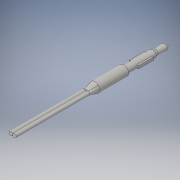
# Autodesk Inventor part: Snap-Twist Idea M
Saved by Autodesk Inventor 2016 (Build 200138000, 138)
## iProperties
Created: 2015-07-29
Part Number: Snap-Twist Idea M
Material: Generic
Document SubType Name: Modeling
Designer: Nancy
Density: 1 g/cm^3
Appearance: Default
Mass: 0.234963 g
Surface Area: 4.60785 cm^2
Volume: 0.234963 cm^3
Author: Nancy
Autodesk Inventor part; units mm, degrees
sketch "Sketch1" plane through (0, 0, 0) normal (0, 0, 1) x (1, 0, 0)
  circle A0 centre (0, 0) radius 0.3405
  dimension "d0" = 0.681
  constraints: 1 centre point, 1 coincident
  measures "d0" diameter of A0
ref_plane "Work Plane1" through (0, 0, 1) normal (0, 0, 1) x (1, 0, 0)
sketch "Sketch2" plane through (0, 0, 1) normal (0, 0, 1) x (1, 0, 0)
  circle A0 centre (0, 0) radius 1.0215
  dimension "d2" = 2.043
  constraints: 1 centre point, 1 coincident
  measures "d2" diameter of A0
ref_plane "Work Plane2" through (0, 0, 4) normal (0, 0, 1) x (1, 0, 0)
sketch "Sketch3" plane through (0, 0, 4) normal (0, 0, 1) x (1, 0, 0)
  circle A0 centre (0, 0) radius 0.8476
  dimension "d4" = 1.6951
  constraints: 1 centre point, 1 coincident
  measures "d4" diameter of A0
ref_plane "Work Plane3" through (0, 0, 5) normal (0, 0, 1) x (1, 0, 0)
sketch "Sketch4" plane through (0, 0, 5) normal (0, 0, 1) x (1, 0, 0)
  circle A0 centre (0, 0) radius 1.1935
  dimension "d6" = 2.387
  constraints: 1 centre point, 1 coincident
  measures "d6" diameter of A0
loft "Loft1" add profiles "Sketch4", "Sketch3"
loft "Loft2" add profiles "Sketch2" section 1 edges at (-0.8476, 0, 4)
loft "Loft3" add profiles "Sketch1" section 2 edges at (-1.0215, 0, 1)
sketch "Sketch5" plane through (0, 0, 5) normal (0, 0, 1) x (1, 0, 0)
  circle A0 centre (0, 0) radius 1.1906
  dimension "d35" = 2.3813
  constraints: 1 centre point, 1 coincident
  measures "d35" diameter of A0
extrude "Extrusion1" add sketch "Sketch5" along normal blind 10
sketch "Sketch6" plane through (0, 0, 15) normal (0, 0, 1) x (1, 0, 0)
  circle A0 centre (0, 0) radius 1.7038
  dimension "d21" = 3.4076
  constraints: 1 centre point, 1 coincident
  measures "d21" diameter of A0
extrude "Extrusion2" add sketch "Sketch6" along normal blind 10
ref_plane "Work Plane4" through (0, 0, 28) normal (0, 0, 1) x (1, 0, 0)
sketch "Sketch7" plane through (0, 0, 28) normal (0, 0, 1) x (1, 0, 0)
  arc A0 (-0.635, 0.635) -> (-0.635, -0.635) centre (-0.635, 0) ccw
  arc A1 (0.635, -0.635) -> (0.635, 0.635) centre (0.635, 0) ccw
  line L0 (-0.635, 0.635) -> (0.635, 0.635)
  line L1 (0.635, -0.635) -> (-0.635, -0.635)
  constraints: 4 end point, 4 point on circle, 2 centre point, 2 tangent
loft "Loft4" add profiles "Sketch7" section 1 edges at (-1.7038, 0, 25)
sketch "Sketch8" plane through (0, 0, 28) normal (0, 0, 1) x (1, 0, 0)
  arc A0 (-0.635, 0.635) -> (-0.635, -0.635) centre (-0.635, 0) ccw projected
  circle A1 centre (-0.635, 0) radius 0.635
  arc A2 (0.635, -0.635) -> (0.635, 0.635) centre (0.635, 0) ccw projected
  circle A3 centre (0.635, 0) radius 0.635
  point P0 (0, 0)
  constraints: 2 coincident, 1 centre point, 1 horizontal alignment, 2 other
extrude "Extrusion3" add sketch "Sketch8" along normal blind 25.4
ref_plane "Work Plane5" through (0, 0, 0) normal (1, 0, 0) x (0, 1, 0)
sketch "Sketch9" plane through (0, 0, 0) normal (1, 0, 0) x (0, 1, 0)
  line L0 (0.508, 11.571) -> (-0.508, 11.571)
  line L1 (-0.508, 11.571) -> (-0.508, 6.27)
  line L2 (-0.508, 6.27) -> (0.508, 6.27)
  line L3 (0.508, 6.27) -> (0.508, 11.571)
  line L4 (-1.7038, 15) -> (1.7038, 15) projected
  line L5 (-1.1935, 5) -> (1.1935, 5) projected
  point P0 (0, 0)
  dimension "d37" = 0.508
  dimension "d38" = 0.508
  dimension "d39" = 3.429
  dimension "d40" = 1.27
  constraints: 8 end point, 2 parallel, 1 horizontal, 1 perpendicular
  measures "d37" distance from line of point (0, 0) L3
  measures "d38" distance from line of point (0, 0) L1
  measures "d39" distance between parallel lines of L4 L0
  measures "d40" distance between parallel lines of L5 L2
extrude "Extrusion4" add sketch "Sketch9" along normal mid plane 3.175
body "Solid1"
